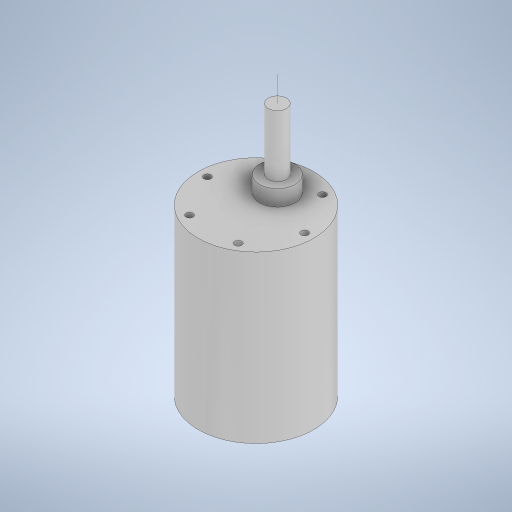
# Autodesk Inventor part: DC 12V 200RPM
Saved by Autodesk Inventor 2024 (Build 280153000, 153)
## iProperties
Created: 2023-10-29
Part Number: DC 12V 200RPM
Material: Generic
Document SubType Name: Modeling
Designer: CJ110
Density: 1 g/cm^3
Appearance: Aluminum - Dark
Mass: 57.321 g
Surface Area: 87.8337 cm^2
Volume: 57.321 cm^3
Author: CJ110
Autodesk Inventor part; units mm, degrees
ref_plane "YZ Plane" through (0, 0, 0) normal (1, 0, 0) x (0, 1, 0)
ref_plane "XZ Plane" through (0, 0, 0) normal (0, 1, 0) x (-1, 0, 0)
ref_plane "XY Plane" through (0, 0, 0) normal (0, 0, 1) x (1, 0, 0)
sketch "Sketch1" plane through (0, 0, 0) normal (0, 1, 0) x (-1, 0, 0)
  circle A0 centre (0, 0) radius 18.415
  dimension "d0" = 36.83
  constraints: 1 centre point, 1 coincident
  measures "d0" diameter of A0
extrude "Extrusion1" add sketch "Sketch1" along normal blind 52.832
sketch "Sketch2" plane through (0, 52.832, 0) normal (0, 1, 0) x (1, 0, 0)
  circle A0 centre (0, 6.8072) radius 5.6642
  line L0 (-18.3795, 1.143) -> (18.3795, 1.143) construction
  circle A1 centre (0, 0) radius 18.415 projected
  line L1 (-28.9381, -18.415) -> (33.3416, -18.415) construction
  circle A2 centre (0, 0) radius 18.415 projected
  dimension "d3" = 11.3284
  dimension "d10" = 19.558
  constraints: 4 end point, 2 horizontal, 2 point on circle, 2 tangent, 1 centre point, 1 vertical alignment
  measures "d3" diameter of A0
  measures "d10" distance between parallel lines of L0 L1
extrude "Extrusion2" add sketch "Sketch2" along normal blind 5.08 contours A0
sketch "Sketch3" plane through (0, 57.912, -6.8072) normal (0, 1, 0) x (1, 0, 0)
  circle A0 centre (0, 0) radius 2.921
  point P0 (0, -6.8072)
  dimension "d6" = 5.842
  constraints: 1 centre point
  measures "d6" diameter of A0
extrude "Extrusion3" add sketch "Sketch3" along normal blind 19.558
sketch "Sketch4" plane through (0, 52.832, 0) normal (0, 1, 0) x (1, 0, 0)
  circle A0 centre (-7.747, 13.4182) radius 1.143
  circle A1 centre (0, 6.8072) radius 5.6642 projected
  circle A2 centre (0, 0) radius 18.415 projected
  circle A3 centre (-15.494, 0) radius 1.143
  circle A4 centre (-7.747, -13.4182) radius 1.143
  circle A5 centre (7.747, -13.4182) radius 1.143
  circle A6 centre (15.494, 0) radius 1.143
  circle A7 centre (7.747, 13.4182) radius 1.143
  circle A8 centre (0, 0) radius 18.415 projected
  line L0 (0, 0) -> (-16.637, 0) construction
  line L1 (-18.415, 3.3425) -> (-18.415, -3.4032) construction
  dimension "d11" = 2.286
  dimension "d14" = 360
  dimension "d16" = 1.778
  constraints: 5 centre point, 4 end point, 2 horizontal alignment, 1 horizontal, 1 perpendicular, 1 tangent, 1 vertical, 15 other
  measures "d11" diameter of A0
  measures "d16" distance from line of L1 L0.end
extrude "Extrusion4" cut sketch "Sketch4" against normal blind 7.62 contours A0 | A3 | A4 | A5 | A6 | A7
body "Solid1"
